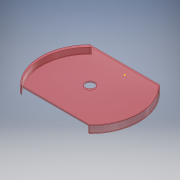
# Autodesk Inventor part: Gear Container
Saved by Autodesk Inventor 2017 (Build 210142000, 142)
## iProperties
Created: 2018-12-12
Part Number: Gear Container
Material: Generic
Document SubType Name: Modeling
Designer: Matt
Density: 1 g/cm^3
Appearance: Dark Red
Mass: 177.976 g
Surface Area: 1028.66 cm^2
Volume: 177.976 cm^3
Author: Matt
Autodesk Inventor part; units mm, degrees
ref_plane "YZ Plane" through (0, 0, 0) normal (1, 0, 0) x (0, 1, 0)
ref_plane "XZ Plane" through (0, 0, 0) normal (0, 1, 0) x (-1, 0, 0)
sketch "Sketch1" plane through (0, 0, 0) normal (0, 0, 1) x (1, 0, 0)
  circle A0 centre (0, 0) radius 130
  dimension "d0" = 260
  constraints: 1 centre point, 1 coincident
  measures "d0" diameter of A0
extrude "Extrusion1" add sketch "Sketch1" along normal blind 24
ref_plane "Work Plane1" through (0, 0, 12) normal (0, 0, 1) x (1, 0, 0)
sketch "Sketch3" plane through (0, 0, 12) normal (0, 0, 1) x (1, 0, 0)
  circle A0 centre (0, 0) radius 127.5
  dimension "d4" = 255
  constraints: 1 centre point, 1 coincident
  measures "d4" diameter of A0
extrude "Extrusion2" cut sketch "Sketch3" along normal mid plane 16.5
sketch "Sketch4" plane through (0, 0, 24) normal (0, 0, 1) x (1, 0, 0)
  circle A0 centre (0, 0) radius 12.5
  dimension "d7" = 25
  constraints: 1 centre point, 1 coincident
  measures "d7" diameter of A0
extrude "Extrusion3" cut sketch "Sketch4" against normal blind 5
sketch "Sketch5" plane through (0, 0, 24) normal (0, 0, 1) x (1, 0, 0)
  line L0 (0, 0) -> (91.9239, 91.9239)
  circle A0 centre (0, 0) radius 130 projected
  line L1 (0, 0) -> (130, 0) construction
  line L2 (91.9239, 91.9239) -> (-91.9239, 91.9239)
  arc A1 (91.9239, 91.9239) -> (-91.9239, 91.9239) centre (0, 0) ccw
  dimension "d10" = 45
  constraints: 6 end point, 4 point on circle, 2 horizontal, 1 centre point, 1 concentric, 1 equal length
  measures "d10" angle of L1 L0
extrude "Extrusion4" cut sketch "Sketch5" against normal through all contours L2 A0 picked at (-17.7846, 107.7382)
mirror "Mirror1" about plane through (0, 0, 0) normal (0, 1, 0) of "Extrusion4"
sketch "Sketch8" plane through (0, 0, 0) normal (0, 0, -1) x (-1, 0, 0)
  line L0 (91.9239, 91.9239) -> (-91.9239, 91.9239) projected
  line L1 (-91.9239, 91.9239) -> (91.9239, 91.9239)
  arc A0 (91.9239, -91.9239) -> (91.9239, 91.9239) centre (0, 0) ccw projected
  arc A1 (91.9239, -91.9239) -> (91.9239, 91.9239) centre (91.9239, 0) ccw
  line L2 (91.9239, -91.9239) -> (-91.9239, -91.9239)
  arc A2 (-91.9239, 91.9239) -> (-91.9239, -91.9239) centre (0, 0) ccw projected
  arc A3 (-91.9239, 91.9239) -> (-91.9239, -91.9239) centre (-91.9239, 0) ccw
  dimension "d15" = 183.8478
  dimension "d16" = 183.8478
  constraints: 4 end point, 4 point on circle, 2 centre point, 1 collinear, 1 horizontal
  measures "d15" distance of L0.start L0.end
  measures "d16" distance between parallel lines of L2 L0
extrude "Extrusion5" cut sketch "Sketch8" against normal blind 3.75
sketch "Sketch9" plane through (-91.9239, 91.9239, 24) normal (0, 1, 0) x (1, 0, 0)
  point P0 (91.9239, 24)
body "Solid1"
